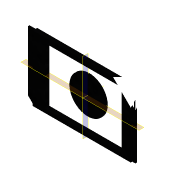
# Autodesk Inventor part: 03_LCD_Frame
Saved by Autodesk Inventor 2016 (Build 200138000, 138)
## iProperties
Created: 2016-11-08
Part Number: 03_LCD_Frame
Material: Generisch
Document SubType Name: Modeling
Designer: Bene
Density: 1 g/cm^3
Appearance: Schwarz
Author: Bene
Autodesk Inventor part; units mm, degrees
ref_plane "YZ Plane" through (0, 0, 0) normal (1, 0, 0) x (0, 1, 0)
ref_plane "XZ Plane" through (0, 0, 0) normal (0, 1, 0) x (-1, 0, 0)
ref_plane "XY Plane" through (0, 0, 0) normal (0, 0, 1) x (1, 0, 0)
sketch "Skizze1" plane through (0, 0, 0) normal (0, 0, 1) x (1, 0, 0)
  circle A0 centre (-20.2101, 34.0775) radius 3.5 projected
  circle A1 centre (16.2899, -67.9225) radius 3.5 projected
  circle A2 centre (27.7899, 31.0775) radius 1.5 projected
  circle A3 centre (-1.7101, -51.9225) radius 1.5 projected
  line L0 (-11.7101, -72.9225) -> (30.2899, -72.9225) projected
  line L1 (30.2899, -72.9225) -> (30.2899, 68.0775) projected
  line L2 (30.2899, 68.0775) -> (-32.7101, 68.0775) projected
  line L3 (-32.7101, 68.0775) -> (-32.7101, -51.9225) projected
  line L4 (-32.7101, -51.9225) -> (-11.7101, -72.9225) projected
  line L5 (24.8394, -0.0171) -> (-45.1606, -0.0171)
  line L6 (-45.1606, -0.0171) -> (-45.1606, -1.0171)
  line L7 (-45.1606, -1.0171) -> (24.8394, -1.0171)
  line L8 (24.8394, -1.0171) -> (24.8394, -0.0171)
  line L9 (22.8394, -1.0171) -> (-41.1606, -1.0171)
  line L10 (-41.1606, -1.0171) -> (-41.1606, -2.0171)
  line L11 (-41.1606, -2.0171) -> (22.8394, -2.0171)
  line L12 (22.8394, -2.0171) -> (22.8394, -1.0171)
  line L13 (22.8394, -0.0171) -> (-41.1606, -0.0171)
  line L14 (-41.1606, -0.0171) -> (-41.1606, 0.9829)
  line L15 (-41.1606, 0.9829) -> (22.8394, 0.9829)
  line L16 (22.8394, 0.9829) -> (22.8394, -0.0171)
  point P0 (0, 0)
  dimension "d0" = 70
  dimension "d1" = 1
  dimension "d2" = 64
  dimension "d3" = 1
  dimension "d4" = 2
  dimension "d5" = 1
  constraints: 24 end point, 6 parallel, 3 horizontal, 3 perpendicular, 2 point on line
  measures "d0" distance of L7.end L6.end
  measures "d1" distance of L6.end L5.end
  measures "d2" distance of L11.end L10.end
  measures "d3" distance of L10.end L9.end
  measures "d4" distance of L9.start L7.end
  measures "d5" distance of L13.end L14.end
extrude "Extrusion1" add sketch "Skizze1" along normal blind 42.5 contours L11 L10 L7 L3 | L3 L7 L12 L11 | L7 L6 L5 L3 | L3 L5 L8 L7 | L15 L16 L5 L3 | L3 L5 L14 L15
sketch "Skizze2" plane through (-41.1606, 0.9829, 0) normal (0, 1, 0) x (1, 0, 0)
  line L0 (64, 0) -> (0, 0) projected
  line L1 (0, 0) -> (0, -42.5) projected
  line L2 (64, -42.5) -> (0, -42.5) projected
  line L3 (64, 0) -> (64, -42.5) projected
  line L4 (58, -39.5) -> (8, -39.5)
  line L5 (8, -39.5) -> (8, -2.5)
  line L6 (8, -2.5) -> (58, -2.5)
  line L7 (58, -2.5) -> (58, -39.5)
  point P0 (41.1606, 0)
  dimension "d8" = 50
  dimension "d9" = 37
  dimension "d10" = 3
  dimension "d11" = 6
  constraints: 8 end point, 2 parallel, 1 horizontal, 1 perpendicular
  measures "d8" distance of L5.end L6.end
  measures "d9" distance of L4.end L5.end
  measures "d10" distance between parallel lines of L4 L2
  measures "d11" distance between parallel lines of L3 L7
extrude "Extrusion2" cut sketch "Skizze2" against normal through all contours L4 L5 L6 L7
ref_plane "Arbeitsebene1" through (-8.1606, 0.9829, 2.5) normal (-1, 0, 0) x (0, 0, 1)
ref_plane "Arbeitsebene2" through (-33.1606, 0.9829, 21) normal (0, 0, 1) x (1, 0, 0)
sketch "Skizze5" plane through (-41.1606, 0.9829, 0) normal (0, 1, 0) x (1, 0, 0)
  line L0 (58, -2.5) -> (58, -39.5) construction
  line L1 (58, -39.5) -> (8, -39.5) construction
  line L2 (8, -39.5) -> (8, -2.5) construction
  line L3 (8, -2.5) -> (58, -2.5) construction
  line L4 (64, 0) -> (0, 0) construction
  line L5 (0, 0) -> (0, -42.5) construction
  line L6 (64, -42.5) -> (0, -42.5) construction
  line L7 (64, 0) -> (64, -42.5) construction
  circle A0 centre (39.5, -21) radius 18.5 construction
  circle A1 centre (26.5, -21) radius 18.5 construction
  ellipse E0 centre (33, -21) end of major axis (58, -21) minor radius 18.5 construction
  circle A2 centre (33, -21) radius 12
  point P0 (41.1606, 0)
  constraints: 6 tangent, 3 centre point, 1 coincident, 2 other
extrude "Extrusion3" add sketch "Skizze5" along normal blind 1
